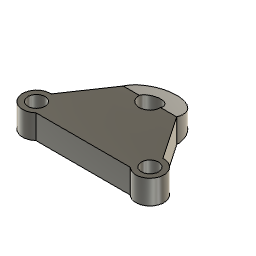
Vernier Camera Mount v4 (Autodesk Fusion 360 design; units mm, degrees)
Autodesk Fusion 360 part; units mm, degrees
sketch "Main Base" plane through (0, 0, 0) normal (0, 0, 1) x (1, 0, 0) in component "Camera Mount"
  circle A0 centre (0, 0) radius 2
  arc A1 (10, 0) -> (-10, 0) centre (0, 0) ccw
  line L0 (-10, 0) -> (-10, -25)
  line L1 (-10, -25) -> (10, -25)
  line L2 (10, -25) -> (10, 0)
  line L3 (10, -20) -> (-10, -20)
  circle A2 centre (0, 0) radius 4
  dimension "d1" = 4
  constraint coincident A0.centre A1.centre
  constraint tangent A1 L0
  constraint vertical L0
  constraint perpendicular L0 L1
  constraint tangent A1 L2
  constraint coincident L2 L3.start
  constraint coincident L0 L3.end
  constraint perpendicular L0 L3
  constraint concentric A0 A2
  measures "d1" diameter of A0
extrude "Extrude1" add sketch "Main Base" along normal blind 2 contours A2 in component "Camera Mount"
extrude "Extrude2" add sketch "Main Base" along normal blind 5 contours A1 L0 L2 L3 | L0 L1 L2 L3 in component "Camera Mount"
sketch "Constraints" plane through (0, 0, 0) normal (1, 0, 0) x (0, 1, 0)
  line L0 (0, 9) -> (15, 9)
  line L1 (15, 9) -> (15, 0)
  line L2 (15, 0) -> (0, 0)
  line L3 (0, 0) -> (-25, 0)
  line L4 (-25, 0) -> (-25, 4)
  line L5 (-25, 4) -> (-55, 4)
  line L6 (-55, 4) -> (-55, 74)
  line L7 (0, 9) -> (-20, 9)
  line L8 (-20, 9) -> (-20, 74)
  dimension "d8" = 9
  dimension "d9" = 25
  constraint coincident L2.end L3.start
  constraint perpendicular L0 L1
  constraint perpendicular L3 L4
  constraint perpendicular L4 L5
  constraint perpendicular L5 L6
  constraint perpendicular L0 L8
  measures "d8" distance of L2.end L0.start
  measures "d9" distance of L2.end L3.end
sketch "Support Legs" plane through (0, 0, 0) normal (0, 0, 1) x (1, 0, 0) in component "Camera Mount"
  line L0 (20, -25) -> (-20, -25)
  line L1 (-20, -25) -> (-20, -45)
  line L2 (20, -25) -> (20, -45)
  line L3 (10, -20) -> (-10, -20)
  line L4 (-10, -20) -> (-25, -20)
  line L5 (-25, -20) -> (-25, -45)
  line L6 (-25, -45) -> (-20, -45)
  line L7 (20, -45) -> (25, -45)
  line L8 (25, -45) -> (25, -20)
  line L9 (25, -20) -> (10, -20)
  constraint perpendicular L0 L1
  constraint perpendicular L0 L2
  constraint perpendicular L3 L5
  constraint perpendicular L1 L6
  constraint perpendicular L2 L7
  constraint perpendicular L7 L8
  constraint perpendicular L8 L9
extrude "Extrude4" add sketch "Support Legs" along normal blind 5 in component "Camera Mount"
chamfer "Chamfer1" distance 15 angle 45 2 edges at (-10, -20, 2.5) (10, -20, 2.5) in component "Camera Mount"
extrude "Extrude6" cut 2 faces at (-23.3333, -45, 1.6667) (21.6667, -45, 1.6667) along direction (0, 1, 0) blind 20 in component "Camera Mount"
sketch "Rod Inclusion" plane through (0, 0, 0) normal (0, 0, 1) x (1, 0, 0) in component "Camera Mount"
  circle A0 centre (0, 0) radius 2
  circle A1 centre (-21.2132, -21.2132) radius 3.2
  circle A2 centre (21.2132, -21.2132) radius 3.2
  circle A3 centre (-21.2132, -21.2132) radius 4.7
  circle A4 centre (21.2132, -21.2132) radius 4.7
  line L0 (0, -25) -> (18.4293, -25)
  line L1 (0, -25) -> (-18.4293, -25)
  arc A5 (10, 0) -> (-10, 0) centre (0, 0) ccw
  line L2 (-21.2132, -16.5132) -> (-10, 0)
  line L3 (10, 0) -> (21.2132, -16.5132)
  dimension "d24" = 4
  dimension "d25" = 30
  dimension "d26" = 30
  dimension "d27" = 6.4
  dimension "d28" = 6.4
  dimension "d29" = 9.4
  dimension "d30" = 9.4
  constraint coincident A0.centre A5.centre
  constraint concentric A1 A3
  constraint concentric A2 A4
  constraint coincident A4 L0.end
  constraint coincident A3 L1.end
  constraint coincident A3 L2.start
  constraint coincident A4 L3.end
  measures "d24" diameter of A0
  measures "d25" distance of A0.centre A2.centre
  measures "d26" distance of A0.centre A1.centre
  measures "d27" diameter of A1
  measures "d28" diameter of A2
  measures "d29" diameter of A3
  measures "d30" diameter of A4
extrude "Extrude7" cut 1 faces at (-0.0996, -17.9963, 5) along direction (0, 0, -1) blind 15 in component "Camera Mount"
extrude "Extrude8" cut 1 faces at (3.311, -0.2981, 2) along direction (0, 0, -1) blind 6 in component "Camera Mount"
extrude "Extrude9" add sketch "Rod Inclusion" along normal blind 9 in component "Camera Mount"
extrude "Extrude10" cut sketch "Main Base" along normal blind 11 from surface at 2 contours A2 in component "Camera Mount"
sketch "Sketch7" plane through (0, 0, 0) normal (0, 0, 1) x (1, 0, 0) in component "Camera Mount"
  line L0 (0, -20) -> (0, 20)
  circle A0 centre (0, 20) radius 40
  constraint vertical L0
  constraint coincident L0.end A0.centre
  constraint coincident L0.start A0
sketch "Sketch8" plane through (0, 0, 0) normal (0, 0, 1) x (1, 0, 0) in component "Camera Mount"
  line L0 (-21.2, -21.2) -> (0.0132, -42.4132)
  line L1 (-21.2, -21.2) -> (8.8, -21.2) construction
  line L2 (0, -25) -> (0.0132, -42.4132)
  dimension "d40" = 45
  dimension "d41" = 30
  constraint horizontal L1
  measures "d40" angle of L0 L1
  measures "d41" distance of L0.start L0.end
sketch "Sketch3" plane through (0, 0, 0) normal (1, 0, 0) x (0, 1, 0)
  line L0 (10, 9) -> (10, 6)
  line L1 (10, 6) -> (0, 9)
  line L2 (0, 9) -> (10, 9)
  constraint vertical L0
  constraint perpendicular L0 L2
extrude "Extrude11" cut sketch "Sketch3" along normal mid plane 50 in component "Camera Mount"
sketch "Sketch4" plane through (0, 0, 9) normal (0, 0, 1) x (-1, 0, 0)
  line L0 (4, 0) -> (10, 0)
  line L1 (10, 0) -> (21.2132, 16.5132)
  arc A0 (21.2132, 16.5132) -> (18.4293, 25) centre (21.2132, 21.2132) ccw
  line L2 (18.4293, 25) -> (-18.4293, 25)
  arc A1 (-18.4293, 25) -> (-21.2132, 16.5132) centre (-21.2132, 21.2132) ccw
  line L3 (-21.2132, 16.5132) -> (-10, 0)
  line L4 (-10, 0) -> (-4, 0)
  arc A2 (4, 0) -> (-4, 0) centre (0, 0) ccw
  circle A3 centre (-21.2132, 21.2132) radius 3.2
  circle A4 centre (21.2132, 21.2132) radius 3.2
  circle A5 centre (-21.2132, 21.2132) radius 5.2
  circle A6 centre (21.2132, 21.2132) radius 5.2
  circle A7 centre (-21.2132, 21.2132) radius 3.2
  circle A8 centre (21.2132, 21.2132) radius 3.2
  dimension "d44" = 10.4
  dimension "d45" = 10.4
  constraint concentric A1 A5
  constraint concentric A0 A6
  constraint concentric A1 A7
  constraint concentric A6 A8
  measures "d44" diameter of A5
  measures "d45" diameter of A6
extrude "Extrude12" add sketch "Sketch4" against normal blind 9 contours L1 A0 L2 A6 | L1 A0 L2 A6 | L2 A1 L3 A5 | L2 A1 L3 A5 in component "Camera Mount"
sketch "Sketch5" plane through (0, 0, 0) normal (0, 0, 1) x (1, 0, 0)
component "Camera Mount" placed x (1, 0, 0) y (0, 1, 0) z (0, 0, 1) at (0, 0, 0)
